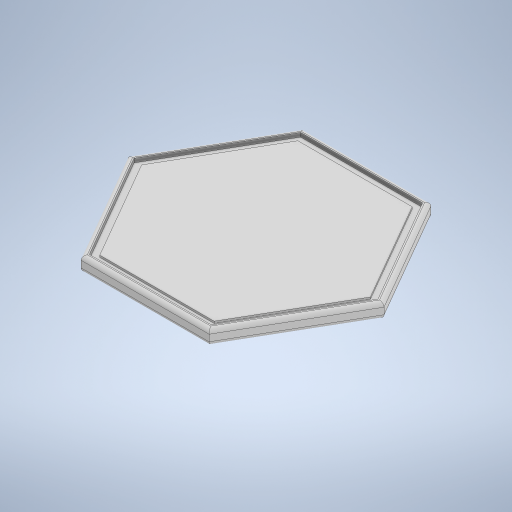
# Autodesk Inventor part: OV-PAM_n_6_bottom
Saved by Autodesk Inventor 2024 (Build 280153000, 153)
## iProperties
Created: 2023-08-31
Part Number: OV-PAM_n_6_bottom
Material: 일반
Document SubType Name: Modeling
Designer: jsw
Density: 1 g/cm^3
Appearance: 기본값
Author: jsw
Autodesk Inventor part; units mm, degrees
ref_plane "YZ Plane" through (0, 0, 0) normal (1, 0, 0) x (0, 1, 0)
ref_plane "XZ Plane" through (0, 0, 0) normal (0, 1, 0) x (-1, 0, 0)
ref_plane "XY Plane" through (0, 0, 0) normal (0, 0, 1) x (1, 0, 0)
sketch "스케치1" plane through (0, 0, 0) normal (0, 1, 0) x (-1, 0, 0)
  line L0 (17.6385, -30.5508) -> (-17.6385, -30.5508)
  line L1 (-17.6385, -30.5508) -> (-35.277, 0)
  line L2 (-35.277, 0) -> (-17.6385, 30.5508)
  line L3 (-17.6385, 30.5508) -> (17.6385, 30.5508)
  line L4 (17.6385, 30.5508) -> (35.277, 0)
  line L5 (35.277, 0) -> (17.6385, -30.5508)
  line L6 (19.486, -33.7508) -> (-19.486, -33.7508)
  line L7 (-19.486, -33.7508) -> (-38.972, 0)
  line L8 (-38.972, 0) -> (-19.486, 33.7508)
  line L9 (-19.486, 33.7508) -> (19.486, 33.7508)
  line L10 (19.486, 33.7508) -> (38.972, 0)
  line L11 (38.972, 0) -> (19.486, -33.7508)
  point P0 (0, 0)
  point P1 (0, 0)
  point P2 (0, 0)
  dimension "d0" = 70.554
  dimension "d1" = 3.2
  constraints: 24 end point, 2 coincident, 2 horizontal, 26 other
  measures "d0" distance of L2.end L0.start
  measures "d1" distance between parallel lines of L0 L6
extrude "돌출1" add sketch "스케치1" along normal blind 4.4 contours L0 L1 L2 L3 L4 L5 | L6 L7 L8 L9 L10 L11
sketch "스케치2" plane through (0, 4.4, 0) normal (0, 1, 0) x (1, 0, 0)
  line L0 (-18.5623, 32.1508) -> (18.5623, 32.1508)
  line L1 (18.5623, 32.1508) -> (37.1245, 0)
  line L2 (37.1245, 0) -> (18.5623, -32.1508)
  line L3 (18.5623, -32.1508) -> (-18.5623, -32.1508)
  line L4 (-18.5623, -32.1508) -> (-37.1245, 0)
  line L5 (-37.1245, 0) -> (-18.5623, 32.1508)
  line L6 (-19.486, 33.7508) -> (-38.972, 0) projected
  point P0 (0, 0)
  point P1 (0, 0)
  dimension "d4" = 1.6
  constraints: 12 end point, 1 coincident, 1 horizontal, 13 other
  measures "d4" distance between parallel lines of L5 L6
extrude "돌출2" cut sketch "스케치2" against normal blind 1.2
sketch "스케치3" plane through (0, 3.2, 0) normal (0, 1, 0) x (1, 0, 0)
  line L0 (17.4076, -30.1508) -> (-17.4076, -30.1508)
  line L1 (-17.4076, -30.1508) -> (-34.8151, 0)
  line L2 (-34.8151, 0) -> (-17.4076, 30.1508)
  line L3 (-17.4076, 30.1508) -> (17.4076, 30.1508)
  line L4 (17.4076, 30.1508) -> (34.8151, 0)
  line L5 (34.8151, 0) -> (17.4076, -30.1508)
  line L6 (-18.5623, 32.1508) -> (18.5623, 32.1508) projected
  point P0 (0, 0)
  point P1 (0, 0)
  dimension "d7" = 2
  constraints: 12 end point, 1 coincident, 1 horizontal, 13 other
  measures "d7" distance between parallel lines of L6 L3
extrude "돌출3" add sketch "스케치3" along normal blind 0.6
fillet "모깎기1" radius 1.2 12 edges at (0, 4.4, -33.7508) (0, 0, -33.7508) (-29.229, 4.4, -16.8754) (-29.229, 0, -16.8754) (-29.229, 4.4, 16.8754) (-29.229, 0, 16.8754) (0, 0, 33.7508) (0, 4.4, 33.7508) (29.229, 0, 16.8754) (29.229, 4.4, 16.8754) (29.229, 4.4, -16.8754) (29.229, 0, -16.8754)
sketch "스케치4" plane through (0, 0, 0) normal (0, -1, 0) x (1, 0, 0)
  line L0 (10, -7.5) -> (-10, -7.5)
  line L1 (-10, -7.5) -> (-10, -2.5)
  line L2 (-10, -2.5) -> (10, -2.5)
  line L3 (10, -2.5) -> (10, -7.5)
  line L4 (10, -7.5) -> (-10, -2.5) construction
  line L5 (-10, -7.5) -> (10, -2.5) construction
  line L6 (10, 2.5) -> (-10, 2.5)
  line L7 (-10, 2.5) -> (-10, 7.5)
  line L8 (-10, 7.5) -> (10, 7.5)
  line L9 (10, 7.5) -> (10, 2.5)
  line L10 (10, 2.5) -> (-10, 7.5) construction
  line L11 (-10, 2.5) -> (10, 7.5) construction
  point P0 (0, 0)
  point P1 (0, -5)
  point P2 (0, 5)
  dimension "d11" = 20
  dimension "d12" = 5
  dimension "d13" = 20
  dimension "d14" = 5
  dimension "d16" = 5
  dimension "d17" = 2.5
  constraints: 24 end point, 4 midpoint, 4 parallel, 2 horizontal, 2 perpendicular, 2 vertical alignment
  measures "d11" distance of L1.end L2.end
  measures "d12" distance of L0.end L1.end
  measures "d13" distance of L7.end L8.end
  measures "d14" distance of L6.end L7.end
  measures "d16" distance between parallel lines of L2 L6
  measures "d17" distance from line of L2 point (0, 0)
extrude "돌출4" add sketch "스케치4" along normal blind 10
sketch "스케치5" plane through (10, 0, -7.5) normal (0, 0, -1) x (-1, 0, 0)
  circle A0 centre (15, -5) radius 1.25
  circle A1 centre (5, -5) radius 1.25
  line L0 (0, 0) -> (0, -10) projected
  line L1 (-8.7932, 0) -> (28.7932, 0) projected
  point P0 (10, 0)
  point P1 (0, -5)
  dimension "d20" = 2.5
  dimension "d21" = 2.5
  dimension "d22" = 5
  dimension "d23" = 5
  dimension "d24" = 10
  constraints: 2 centre point, 1 horizontal alignment, 1 midpoint
  measures "d20" diameter of A0
  measures "d21" diameter of A1
  measures "d22" distance of A1.centre point (0, -5)
  measures "d23" distance from line of L1 A1.centre
  measures "d24" distance of A0.centre A1.centre
extrude "돌출5" cut sketch "스케치5" against normal up to surface (15 mm away)
equation "\"d17\" = 0.5 * d16"
